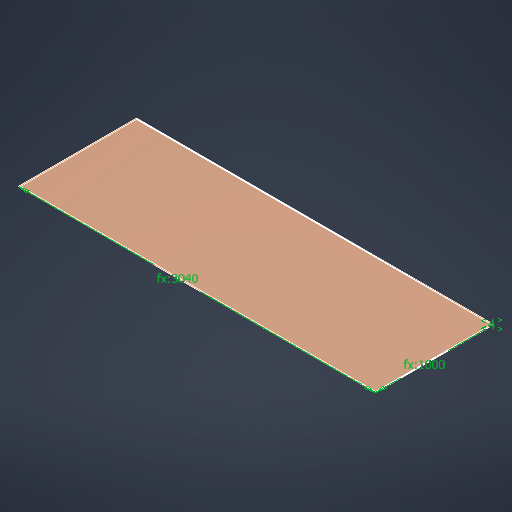
# Autodesk Inventor part: CONVEYOR SURFACE-01
Saved by Autodesk Inventor 2025 (Build 290162000, 162)
## iProperties
Created: 2024-05-06
Part Number: CONVEYOR SURFACE-01
Material: Generic
Document SubType Name: Modeling
Designer: zulet
Density: 1 g/cm^3
Appearance: Default
Author: zulet
Autodesk Inventor part; units mm, degrees
ref_plane "YZ Plane" through (0, 0, 0) normal (1, 0, 0) x (0, 1, 0)
ref_plane "XZ Plane" through (0, 0, 0) normal (0, 1, 0) x (-1, 0, 0)
ref_plane "XY Plane" through (0, 0, 0) normal (0, 0, 1) x (1, 0, 0)
sketch "Sketch1" plane through (0, 0, 0) normal (0, 1, 0) x (-1, 0, 0)
  line L0 (0, 0) -> (3040, 0)
  line L1 (3040, 0) -> (3040, -1000)
  line L2 (3040, -1000) -> (0, -1000)
  line L3 (0, -1000) -> (0, 0)
  line L4 (0, -1000) -> (4, -1000)
  line L5 (4, -1000) -> (4, -996)
  line L6 (4, -996) -> (0, -996)
  line L7 (0, -996) -> (0, -1000)
  point P0 (0, -996)
  dimension "d0" = 1000
  dimension "d1" = 3040
  dimension "d3" = 4
  dimension "d4" = 4
  constraints: 16 end point, 4 parallel, 2 horizontal, 2 perpendicular
  measures "d0" distance of L2.end L0.start
  measures "d1" distance of L0.start L0.end
  measures "d3" distance of L6.end L5.end
  measures "d4" distance of L5.end L4.end
boundary_patch "Boundary Patch1"
extrude "Extrusion1" add sketch "Sketch1" against normal blind 4 contours L6 L5 L2 L3
equation "\"d0\" = conveyorWidth"
equation "\"d1\" = conveyorLength"
equation "\"conveyorWidth\" = 1000"
equation "\"conveyorLength\" = 3040"
body "Solid1"
body "Srf1"
